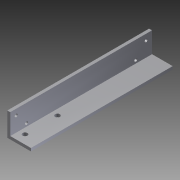
# Autodesk Inventor part: 8 ball corner L
Saved by Autodesk Inventor 2012 (Build 160160000, 160)
## iProperties
Created: 2013-10-10
Part Number: 8 ball corner L
Material: Default
Document SubType Name: Modeling
Designer: Bryce
Density: 1 g/cm^3
Author: Bryce
Autodesk Inventor part; units mm, degrees
ref_plane "YZ Plane" through (0, 0, 0) normal (1, 0, 0) x (0, 1, 0)
ref_plane "XZ Plane" through (0, 0, 0) normal (0, 1, 0) x (-1, 0, 0)
ref_plane "XY Plane" through (0, 0, 0) normal (0, 0, 1) x (1, 0, 0)
sketch "Sketch1" plane through (0, 0, 0) normal (0, 0, 1) x (1, 0, 0)
  line L0 (0, 0) -> (25.4, 0)
  line L1 (25.4, 0) -> (25.4, 3.175)
  line L2 (3.175, 25.4) -> (0, 25.4)
  line L3 (0, 25.4) -> (0, 0)
  line L4 (3.175, 25.4) -> (3.175, 3.175)
  line L5 (3.175, 3.175) -> (25.4, 3.175)
  dimension "d0" = 25.4
  dimension "d1" = 25.4
  dimension "d2" = 3.175
  dimension "d3" = 3.175
  constraints: 12 end point, 2 parallel, 1 horizontal, 1 perpendicular
  measures "d0" distance of L0.start L0.end
  measures "d1" distance of L2.end L0.start
  measures "d2" distance between parallel lines of L3 L4
  measures "d3" distance between parallel lines of L0 L5
extrude "Extrusion1" add sketch "Sketch1" along normal blind 152.4
sketch "Sketch3" plane through (0, 0, 0) normal (0, -1, 0) x (1, 0, 0)
  line L0 (25.4, 152.4) -> (0, 152.4) projected
  line L1 (0, 0) -> (0, 152.4) projected
  circle A0 centre (9.525, 107.95) radius 2.54
  circle A1 centre (9.525, 142.875) radius 2.54
  dimension "d20" = 9.525
  dimension "d21" = 34.925
  dimension "d22" = 5.08
  dimension "d23" = 9.525
  constraints: 2 centre point, 1 equal radius, 1 vertical alignment
  measures "d20" distance from line of L0 A1.centre
  measures "d21" distance of A1.centre A0.centre
  measures "d22" diameter of A1
  measures "d23" distance from line of A1.centre L1
extrude "Extrusion4" cut sketch "Sketch3" against normal blind 25.4
sketch "Sketch4" plane through (0, 0, 0) normal (-1, 0, 0) x (0, 0, 1)
  line L0 (0, 25.4) -> (0, 0) projected
  line L1 (0, 0) -> (152.4, 0) projected
  circle A0 centre (6.35, 19.05) radius 1.5875
  circle A1 centre (17.4625, 6.35) radius 1.5875
  line L2 (0, 25.4) -> (152.4, 25.4) projected
  line L3 (76.2, 25.4) -> (76.2, 0)
  circle A2 centre (146.05, 19.05) radius 1.5875
  circle A3 centre (134.9375, 6.35) radius 1.5875
  dimension "d26" = 6.35
  dimension "d27" = 19.05
  dimension "d28" = 3.175
  dimension "d29" = 6.35
  dimension "d30" = 17.4625
  constraints: 4 centre point, 2 end point, 2 midpoint, 2 symmetric about line, 1 equal radius, 2 other
  measures "d26" distance from line of L1 A1.centre
  measures "d27" distance from line of L1 A0.centre
  measures "d28" diameter of A0
  measures "d29" distance from line of L0 A0.centre
  measures "d30" distance from line of L0 A1.centre
extrude "Extrusion5" cut sketch "Sketch4" against normal blind 25.4 contours A0 | A1 | A2 | A3
equation "\"d2\" = d3"
body "Solid1"
